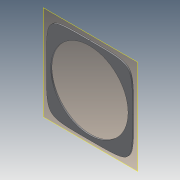
# Autodesk Inventor part: Frame Lower
Saved by Autodesk Inventor 2014 SP1 (Build 180222100, 222)
## iProperties
Created: 2014-04-02
Part Number: Frame Lower
Material: Generic
Document SubType Name: Modeling
Designer: tom
Density: 1 g/cm^3
Appearance: Default
Author: tom
Autodesk Inventor part; units mm, degrees
ref_plane "YZ Plane" through (0, 0, 0) normal (1, 0, 0) x (0, 1, 0)
ref_plane "XZ Plane" through (0, 0, 0) normal (0, 1, 0) x (-1, 0, 0)
ref_plane "XY Plane" through (0, 0, 0) normal (0, 0, 1) x (1, 0, 0)
ref_plane "Work Plane1" through (-138.8109, 23.0767, 114.3) normal (0, 0, 1) x (1, 0, 0)
sketch "Sketch1" plane through (-138.8109, 23.0767, 114.3) normal (0, 0, 1) x (1, 0, 0)
  spline S0 degree 4 poles (0, 95.25) (-76.2, 95.25) (-95.25, 95.25) (-95.25, 76.2) (-95.25, 0) knots 1 1 1 1 1 2 2 2 2 2 projected
  spline S1 degree 4 poles (95.25, 0) (95.25, 76.2) (95.25, 95.25) (76.2, 95.25) (0, 95.25) knots 1 1 1 1 1 2 2 2 2 2 projected
  spline S2 degree 4 poles (0, -95.25) (76.2, -95.25) (95.25, -95.25) (95.25, -76.2) (95.25, 0) knots 1 1 1 1 1 2 2 2 2 2 projected
  spline S3 degree 4 poles (-95.25, 0) (-95.25, -76.2) (-95.25, -95.25) (-76.2, -95.25) (0, -95.25) knots 1 1 1 1 1 2 2 2 2 2 projected
  line L0 (0, 95.25) -> (0, -95.25) construction
  line L1 (95.25, 0) -> (-95.25, 0) construction
  spline S4 degree 3 poles (-93.6625, 0) (-93.6625, 13.1515) (-93.6641, 24.3836) (-93.4921, 34.0057) (-93.1277, 54.3921) (-91.9513, 67.5764) (-88.2745, 76.0527) (-86.2377, 80.7481) (-83.4985, 84.0104) (-79.5283, 86.4707) (-74.4505, 89.6173) (-67.2348, 91.4109) (-56.937, 92.4035) (-43.6826, 93.6811) (-25.4087, 93.6625) (0, 93.6625) knots -2 -2 -2 -2 -1.870556 -1.870556 -1.870556 -1.596305 -1.596305 -1.596305 -1.444385 -1.444385 -1.444385 -1.250085 -1.250085 -1.250085 -1 -1 -1 -1 construction
  spline S5 degree 3 poles (0, 93.6625) (13.1515, 93.6625) (24.3836, 93.6642) (34.0057, 93.4922) (54.392, 93.1278) (67.5764, 91.9513) (76.0526, 88.2745) (80.748, 86.2378) (84.0104, 83.4986) (86.4706, 79.5283) (89.6173, 74.4505) (91.4109, 67.2348) (92.4035, 56.937) (93.681, 43.6826) (93.6625, 25.4087) (93.6625, 0) knots -2 -2 -2 -2 -1.870556 -1.870556 -1.870556 -1.596305 -1.596305 -1.596305 -1.444385 -1.444385 -1.444385 -1.250085 -1.250085 -1.250085 -1 -1 -1 -1 construction
  spline S6 degree 3 poles (0, -93.6625) (-13.1515, -93.6625) (-24.3836, -93.6641) (-34.0057, -93.4921) (-54.392, -93.1277) (-67.5764, -91.9512) (-76.0526, -88.2744) (-80.748, -86.2377) (-84.0104, -83.4985) (-86.4706, -79.5283) (-89.6173, -74.4505) (-91.4109, -67.2347) (-92.4035, -56.9369) (-93.681, -43.6826) (-93.6625, -25.4086) (-93.6625, 0) knots -2 -2 -2 -2 -1.870556 -1.870556 -1.870556 -1.596305 -1.596305 -1.596305 -1.444385 -1.444385 -1.444385 -1.250085 -1.250085 -1.250085 -1 -1 -1 -1 construction
  spline S7 degree 3 poles (93.6625, 0) (93.6625, -13.1514) (93.6641, -24.3836) (93.4921, -34.0057) (93.1277, -54.392) (91.9513, -67.5763) (88.2745, -76.0526) (86.2377, -80.748) (83.4985, -84.0103) (79.5283, -86.4706) (74.4505, -89.6172) (67.2348, -91.4108) (56.937, -92.4034) (43.6826, -93.681) (25.4087, -93.6625) (0, -93.6625) knots -2 -2 -2 -2 -1.870556 -1.870556 -1.870556 -1.596305 -1.596305 -1.596305 -1.444385 -1.444385 -1.444385 -1.250085 -1.250085 -1.250085 -1 -1 -1 -1 construction
  line L2 (-63.5, 63.5) -> (63.5, 63.5) construction
  line L3 (63.5, 63.5) -> (63.5, -63.5) construction
  line L4 (63.5, -63.5) -> (-63.5, -63.5) construction
  line L5 (-63.5, -63.5) -> (-63.5, 63.5) construction
  circle A0 centre (0, 0) radius 85.725
  point P0 (138.8109, -23.0767)
  dimension "d0" = 127
  dimension "d1" = 127
  dimension "d2" = 63.5
  dimension "d3" = 63.5
  dimension "d4" = 171.45
  constraints: 12 end point, 2 parallel, 2 perpendicular, 1 centre point, 1 horizontal, 1 midpoint, 1 vertical
  measures "d0" distance of L3.end L4.end
  measures "d1" distance of L2.end L3.end
  measures "d2" distance between parallel lines of L5 L0
  measures "d3" distance between parallel lines of L2 L1
  measures "d4" diameter of A0
extrude "Extrusion1" add sketch "Sketch1" along normal blind 2.75
body "Solid1"
